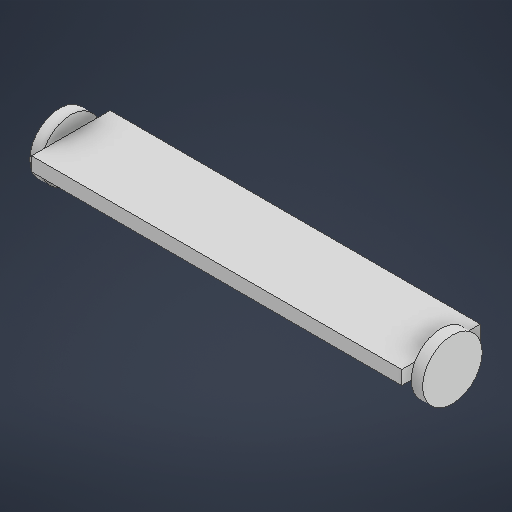
# Autodesk Inventor part: Solor Cleaner - Solor Panal Bace
Saved by Autodesk Inventor 2026 (Build 300175050, 175E)
## iProperties
Created: 2026-02-09
Part Number: Solor Cleaner - Solor Panal Bace
Material: Generic
Document SubType Name: Modeling
Designer: 268021
Density: 1 g/cm^3
Appearance: Default
Author: 268021
Autodesk Inventor part; units mm, degrees
ref_plane "YZ Plane" through (0, 0, 0) normal (1, 0, 0) x (0, 1, 0)
ref_plane "XZ Plane" through (0, 0, 0) normal (0, 1, 0) x (-1, 0, 0)
ref_plane "XY Plane" through (0, 0, 0) normal (0, 0, 1) x (1, 0, 0)
sketch "Sketch1" plane through (0, 0, 0) normal (0, 1, 0) x (-1, 0, 0)
  line L0 (0, 0) -> (-2032, 0)
  line L1 (-2032, 0) -> (-2032, 431.8)
  line L2 (-2032, 431.8) -> (0, 431.8)
  line L3 (0, 431.8) -> (0, 0)
  dimension "d0" = 2032
  dimension "d1" = 431.8
  constraints: 8 end point, 2 parallel, 1 horizontal, 1 perpendicular
  measures "d0" distance of L1.end L2.end
  measures "d1" distance of L0.end L1.end
extrude "Extrusion1" add sketch "Sketch1" along normal blind 76.2
sketch "Sketch2" plane through (0, 0, 0) normal (0, -1, 0) x (1, 0, 0)
  line L0 (2094.0877, 379.5522) -> (2032, 379.5522)
  line L1 (2032, 0) -> (0, 0) projected
  line L2 (0, 431.8) -> (2032, 431.8) projected
  line L3 (-62.0877, 379.5522) -> (0, 379.5522)
  line L4 (2094.0877, 215.9061) -> (2032, 215.9061)
  line L5 (0, 215.9) -> (-62.0877, 215.9061)
  line L6 (2094.0877, 379.5522) -> (2094.0877, 215.9061)
  line L7 (2032, 215.9061) -> (2032, 379.5522)
  line L8 (2032, 431.8) -> (2032, 0) projected
  line L9 (0, 215.9) -> (0, 379.5522)
  line L10 (0, 0) -> (0, 431.8) projected
  line L11 (-62.0877, 215.9061) -> (-62.0877, 379.5522)
  point P0 (2063.0438, 379.5522)
  constraints: 16 end point, 2 collinear, 1 midpoint, 1 perpendicular, 1 vertical
revolve "Revolution1" add sketch "Sketch2" angle 360 about axis through (2094.0877, 0, 215.9061) along (-1, 0, 0) contours L6 L4 L7 L0
sketch "Sketch3" plane through (0, 0, 0) normal (0, -1, 0) x (1, 0, 0)
  line L0 (0, 215.9) -> (-62.0776, 215.9)
  line L1 (0, 431.8) -> (2032, 431.8) projected
  line L2 (0, 431.8) -> (0, 379.5522)
  line L3 (0, 215.9) -> (0, 379.5522)
  line L4 (-62.0776, 215.9) -> (-62.0776, 379.5522)
  line L5 (-62.0776, 379.5522) -> (0, 379.5522)
  point P0 (-31.0388, 431.8)
  dimension "d7" = 62.0776
  dimension "d10" = 215.9
  constraints: 10 end point, 1 horizontal, 1 perpendicular
  measures "d7" distance of L0.start L0.end
  measures "d10" distance from line of L0 point (-31.039, 431.8)
revolve "Revolution2" add sketch "Sketch3" angle 360 about axis through (0, 0, 215.9) along (-1, 0, 0)
body "Solid1"
